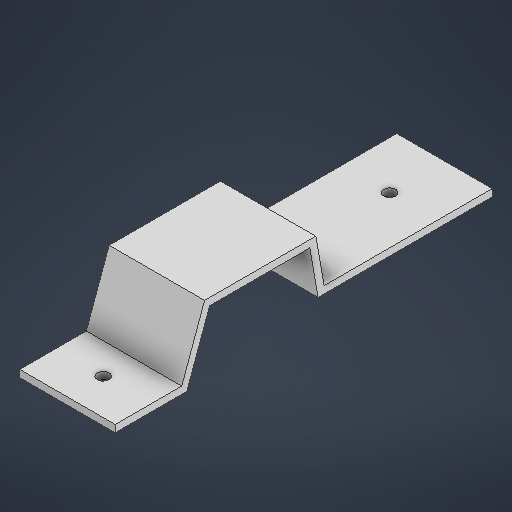
# Autodesk Inventor part: 1.2.3.UpperArmLink1
Saved by Autodesk Inventor 2026.1 (Build 301233020, 233B)
## iProperties
Created: 2025-10-08
Part Number: 1.2.3.UpperArmLink1
Material: Genérico
Document SubType Name: Modeling
Designer: vitos
Density: 1 g/cm^3
Appearance: Valor por defecto
Author: vitos
Autodesk Inventor part; units mm, degrees
ref_plane "YZ Plane" through (0, 0, 0) normal (1, 0, 0) x (0, 1, 0)
ref_plane "XZ Plane" through (0, 0, 0) normal (0, 1, 0) x (-1, 0, 0)
ref_plane "XY Plane" through (0, 0, 0) normal (0, 0, 1) x (1, 0, 0)
sketch "Boceto1" plane through (0, 0, 0) normal (1, 0, 0) x (0, 1, 0)
  line L0 (3, 30) -> (0, 30)
  line L1 (0, 30) -> (0, 0)
  line L2 (0, 0) -> (26.3114, -9.5766)
  line L3 (0, 0) -> (28, 0) construction
  line L4 (26.3114, -9.5766) -> (26.3114, -51.5766)
  line L5 (26.3114, -51.5766) -> (6.6152, -55.0495)
  line L6 (6.6152, -55.0495) -> (6.6152, -128.0495)
  line L7 (6.6152, -128.0495) -> (9.6152, -128.0495)
  line L8 (9.6152, -128.0495) -> (9.6152, -57.5668)
  line L9 (6.6152, -55.0495) -> (6.6152, -58.0495)
  line L10 (29.3114, -9.5766) -> (29.3114, -54.0939)
  line L11 (27.3375, -6.7575) -> (3, 2.1006)
  line L12 (3, 2.1006) -> (3, 30)
  line L13 (29.3114, -54.0939) -> (9.6152, -57.5668)
  line L14 (27.3375, -6.7575) -> (29.3114, -7.4759)
  line L15 (29.3114, -9.5766) -> (29.3114, -7.4759)
  dimension "d0" = 3
  dimension "d2" = 28
  dimension "d3" = 20
  dimension "d6" = 100
  dimension "d7" = 73
  dimension "d8" = 3
  dimension "d9" = 3
  dimension "d12" = 3
  dimension "d13" = 3
  constraints: 32 end point, 2 parallel, 2 perpendicular, 2 vertical, 1 collinear, 1 equal length, 1 horizontal, 1 point on line
  measures "d0" distance of L0.end L0.start
  measures "d2" distance of L1.end L2.end
  measures "d3" angle of L2 L3
  measures "d6" angle of L4 L5
  measures "d7" distance of L5.end L6.end
  measures "d8" distance of L6.end L7.end
  measures "d9" distance of L5.end L9.end
  measures "d12" distance of L2.end L11.start
  measures "d13" distance of L2.end L10.start
extrude "Extrusión1" add sketch "Boceto1" along normal blind 40
sketch "Boceto2" plane through (0, 0, 0) normal (0, -1, 0) x (1, 0, 0)
  circle A0 centre (20, 15) radius 2.5
  point P0 (0, 0)
  dimension "d16" = 5
  constraints: 1 centre point
  measures "d16" diameter of A0
extrude "Extrusión2" cut sketch "Boceto2" against normal blind 3
sketch "Boceto3" plane through (0, 6.6152, -128.0495) normal (0, -1, 0) x (1, 0, 0)
  circle A0 centre (20, 23) radius 2.5
  point P0 (0, 128.0495)
  dimension "d19" = 5
  constraints: 1 centre point
  measures "d19" diameter of A0
extrude "Extrusión3" cut sketch "Boceto3" against normal blind 3
